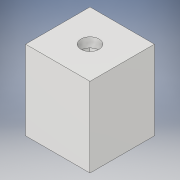
# Autodesk Inventor part: Sample 1x1 tall
Saved by Autodesk Inventor 2018 (Build 220112000, 112)
## iProperties
Created: 2018-05-04
Part Number: Sample 1x1 tall
Material: ABS Plastic
Document SubType Name: Modeling
Designer: Kyle
Density: 1.06 g/cm^3
Appearance: Smooth - White
Author: Kyle
Autodesk Inventor part; units mm, degrees
ref_plane "YZ Plane" through (0, 0, 0) normal (1, 0, 0) x (0, 1, 0)
ref_plane "XZ Plane" through (0, 0, 0) normal (0, 1, 0) x (-1, 0, 0)
ref_plane "XY Plane" through (0, 0, 0) normal (0, 0, 1) x (1, 0, 0)
sketch "Sketch1" plane through (0, 0, 0) normal (0, 1, 0) x (-1, 0, 0)
  line L0 (0, 0) -> (-7.7978, 0)
  line L1 (-7.7978, 0) -> (-7.7978, -7.7978)
  line L2 (-7.7978, -7.7978) -> (0, -7.7978)
  line L3 (0, -7.7978) -> (0, 0)
  dimension "d0" = 7.7978
  dimension "d1" = 7.7978
  constraints: 8 end point, 2 parallel, 1 horizontal, 1 perpendicular
  measures "d0" distance of L2.end L1.end
  measures "d1" distance of L1.end L0.end
extrude "Extrusion1" add sketch "Sketch1" along normal blind 9.6088
shell "Shell1" thickness 1.4732 removed faces 1 at (5.1985, 0, -2.5993)
sketch "Sketch2" plane through (1.4732, 8.1356, -1.4732) normal (0, -1, 0) x (1, 0, 0)
  line L0 (0, -4.8514) -> (0, 0) projected
  line L1 (4.8514, 0) -> (4.8514, -4.8514) projected
  line L2 (0, 0) -> (4.8514, 0)
  line L3 (4.8514, 0) -> (4.8514, -4.8514)
  line L4 (4.8514, -4.8514) -> (0, -4.8514)
  line L5 (0, -4.8514) -> (0, 0)
  point P0 (-1.4732, 1.4732)
  constraints: 8 end point, 2 parallel, 1 horizontal, 1 perpendicular
extrude "Extrusion2" cut sketch "Sketch2" against normal blind 0.3048
sketch "Sketch3" plane through (1.4732, 8.4404, -1.4732) normal (0, -1, 0) x (1, 0, 0)
  line L0 (0, 0) -> (4.8514, 0) construction
  line L1 (4.8514, 0) -> (4.8514, -4.8514) construction
  line L2 (4.8514, -4.8514) -> (0, -4.8514) construction
  line L3 (0, -4.8514) -> (0, 0) construction
  line L4 (0, -4.8514) -> (0, 0) construction
  line L5 (0, -2.4257) -> (4.8514, -2.4257) construction
  line L6 (0, 0) -> (4.8514, 0) construction
  line L7 (2.4257, 0) -> (2.4257, -4.8514) construction
  circle A0 centre (2.4257, -2.4257) radius 1.0935
  point P0 (-1.4732, 1.4732)
  dimension "d7" = 2.1869
  constraints: 12 end point, 5 midpoint, 2 parallel, 1 centre point, 1 horizontal, 1 perpendicular
  measures "d7" diameter of A0
extrude "Extrusion3" cut sketch "Sketch3" against normal blind 1.27
body "Solid1"
